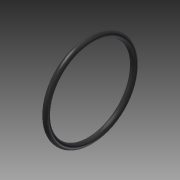
# Autodesk Inventor part: gomu
Saved by Autodesk Inventor 2015 (Build 190159000, 159)
## iProperties
Created: 2013-10-28
Part Number: gomu
Material: 一般
Document SubType Name: Modeling
Designer: kenta
Density: 1 g/cm^3
Appearance: ゴム - 黒 - バージョン 1.1
Mass: 1.06592 g
Surface Area: 14.2122 cm^2
Volume: 1.06592 cm^3
Author: kenta
Autodesk Inventor part; units mm, degrees
ref_plane "YZ Plane" through (0, 0, 0) normal (1, 0, 0) x (0, 1, 0)
ref_plane "XZ Plane" through (0, 0, 0) normal (0, 1, 0) x (-1, 0, 0)
ref_plane "XY Plane" through (0, 0, 0) normal (0, 0, 1) x (1, 0, 0)
sketch "スケッチ1" plane through (0, 0, 0) normal (0, 0, 1) x (1, 0, 0)
  line L0 (-13.0674, 7.7528) -> (-13.0674, -16.2472)
  line L1 (-13.0674, -16.2472) -> (-18.0674, -16.2472)
  line L2 (-18.0674, -16.2472) -> (-18.0674, 7.7528)
  circle A0 centre (-15.5674, 7.7528) radius 1.5
  line L3 (-18.0674, 7.7528) -> (-17.0674, 7.7528)
  line L4 (-14.0674, 7.7528) -> (-13.0674, 7.7528)
  point P0 (0, 0)
  dimension "d2" = 5
  dimension "d3" = 3
  constraints: 10 end point, 3 parallel, 2 horizontal, 2 perpendicular, 2 point on circle, 1 centre point
  measures "d2" distance between parallel lines of L2 L0
  measures "d3" diameter of A0
revolve "回転1" add sketch "スケッチ1" angle 360 about axis through (-13.0674, -16.2472, 0) along (-1, 0, 0) contours A0
